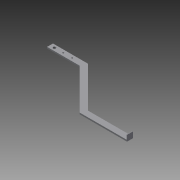
# Autodesk Inventor part: Z-PickupArm-L
Saved by Autodesk Inventor 2013 (Build 170138000, 138)
## iProperties
Created: 2014-01-22
Part Number: Z-PickupArm-L
Material: Generic
Document SubType Name: Modeling
Designer: Jarod
Density: 1 g/cm^3
Author: Jarod
Autodesk Inventor part; units mm, degrees
ref_plane "YZ Plane" through (0, 0, 0) normal (1, 0, 0) x (0, 1, 0)
ref_plane "XZ Plane" through (0, 0, 0) normal (0, 1, 0) x (-1, 0, 0)
ref_plane "XY Plane" through (0, 0, 0) normal (0, 0, 1) x (1, 0, 0)
sketch "Sketch1" plane through (0, 0, 0) normal (0, 1, 0) x (-1, 0, 0)
  line L0 (0, 0) -> (-133.35, 0)
  line L1 (-133.35, 0) -> (-133.35, 25.4)
  line L2 (-133.35, 25.4) -> (0, 25.4)
  line L3 (0, 25.4) -> (0, 0)
  line L4 (-133.35, 25.4) -> (-143.871, 0)
  line L5 (-133.35, 25.4) -> (-105.8572, 25.4) construction
  line L6 (-133.35, 25.4) -> (-151.3105, 7.4395)
  line L7 (-133.35, 25.4) -> (-107.95, 25.4) construction
  line L8 (-151.3105, 7.4395) -> (-143.871, 0)
  line L9 (-133.35, 25.4) -> (-151.3105, 7.4395)
  line L10 (-151.3105, 7.4395) -> (-318.9899, 175.1188)
  line L11 (-318.9899, 175.1188) -> (-301.0293, 193.0793)
  line L12 (-301.0293, 193.0793) -> (-133.35, 25.4)
  circle A0 centre (-12.7, 12.7) radius 6.35
  line L13 (-318.9899, 175.1188) -> (-511.6743, 175.1188)
  line L14 (-511.6743, 175.1188) -> (-511.6743, 200.5188)
  line L15 (-511.6743, 200.5188) -> (-318.9899, 200.5188)
  line L16 (-318.9899, 200.5188) -> (-318.9899, 175.1188)
  line L17 (-318.9899, 175.1188) -> (-308.4688, 200.5188)
  line L18 (-308.4688, 200.5188) -> (-318.9899, 200.5188)
  line L19 (-308.4688, 200.5188) -> (-301.0293, 193.0793)
  line L20 (-133.35, 0) -> (-143.871, 0)
  dimension "d0" = 133.35
  dimension "d1" = 25.4
  dimension "d2" = 112.5
  dimension "d3" = 25.4
  dimension "d4" = 135
  dimension "d5" = 237.1344
  dimension "d6" = 12.7
  dimension "d7" = 192.6844
  dimension "d8" = 25.4
  constraints: 42 end point, 7 parallel, 6 perpendicular, 4 horizontal, 2 equal length, 1 centre point
  measures "d0" distance of L1.end L2.end
  measures "d1" distance of L0.end L1.end
  measures "d2" angle of L4 L5
  measures "d3" distance of L1.end L6.end
  measures "d4" angle of L6 L7
  measures "d5" distance of L6.end L10.end
  measures "d6" diameter of A0
  measures "d7" distance of L14.end L15.end
  measures "d8" distance of L13.end L14.end
extrude "Extrusion1" add sketch "Sketch1" along normal blind 6.35
sketch "Sketch2" plane through (511.6743, 0, 200.5188) normal (1, 0, 0) x (0, 0, -1)
  line L0 (0, 6.35) -> (25.4, 6.35)
  line L1 (25.4, 0) -> (0, 0)
  line L2 (0, 0) -> (0, 25.4)
  line L3 (0, 25.4) -> (25.4, 25.4)
  line L4 (25.4, 25.4) -> (25.4, 0)
  point P0 (200.5188, 0)
  dimension "d15" = 25.4
  dimension "d16" = 25.4
  constraints: 10 end point, 2 horizontal, 2 parallel, 1 perpendicular
  measures "d15" distance of L2.end L3.end
  measures "d16" distance of L1.end L2.end
extrude "Extrusion2" add sketch "Sketch2" along normal blind 1.5875
sketch "Sketch3" plane through (0, 0, 0) normal (-1, 0, 0) x (0, 0, 1)
  line L0 (0, 0) -> (25.4, 0) projected
  line L1 (25.4, 0) -> (25.4, 6.35) projected
  line L2 (0, 6.35) -> (25.4, 6.35) projected
  line L3 (0, 0) -> (0, 6.35) projected
extrude "Extrusion3" add sketch "Sketch3" along normal blind 44.45
sketch "Sketch5" plane through (0, 6.35, 0) normal (0, 1, 0) x (1, 0, 0)
  circle A0 centre (12.7, -12.7) radius 6.35 projected
  line L0 (511.6743, -175.1188) -> (318.9899, -175.1188) projected
  line L1 (12.7, -12.7) -> (12.7, -6.35)
  line L2 (16.3662, -6.35) -> (20.0323, -12.7)
  line L3 (20.0323, -12.7) -> (16.3662, -19.05)
  line L4 (16.3662, -19.05) -> (9.0338, -19.05)
  line L5 (9.0338, -19.05) -> (5.3677, -12.7)
  line L6 (5.3677, -12.7) -> (9.0338, -6.35)
  line L7 (9.0338, -6.35) -> (16.3662, -6.35)
  point P0 (0, 0)
  constraints: 14 end point, 1 coincident, 1 midpoint, 1 perpendicular, 1 vertical alignment, 14 other
extrude "Extrusion5" cut sketch "Sketch5" against normal blind 6.35 contours A0 L2 L3 | A0 L7 L2 | L3 L4 A0 | A0 L6 L7 | L4 L5 A0 | A0 L5 L6
sketch "Sketch7" plane through (0, 6.35, 0) normal (0, 1, 0) x (1, 0, 0)
  line L0 (-44.45, -25.4) -> (-44.45, 0) projected
  line L1 (511.6743, -175.1188) -> (318.9899, -175.1188) projected
  line L2 (-44.45, -12.7) -> (12.7, -12.7)
  line L3 (12.7, -12.7) -> (-25.4, -12.7)
  line L4 (12.7, -12.7) -> (50.8, -12.7) construction
  line L5 (-25.4, -12.7) -> (50.8, -12.7)
  circle A0 centre (-25.4, -12.7) radius 3.175
  circle A1 centre (50.8, -12.7) radius 3.175
  point P0 (0, 0)
  dimension "d31" = 38.1
  dimension "d32" = 180
  dimension "d33" = 76.2
  dimension "d34" = 0
  dimension "d35" = 6.35
  dimension "d36" = 6.35
  constraints: 8 end point, 3 collinear, 2 centre point, 2 coincident, 1 horizontal, 1 midpoint, 1 parallel
  measures "d31" distance of L2.end L3.end
  measures "d32" angle of L3 L4
  measures "d33" distance of L3.end L5.end
  measures "d34" distance between parallel lines of L5 L3
  measures "d35" diameter of A0
  measures "d36" diameter of A1
extrude "Extrusion7" cut sketch "Sketch7" against normal blind 25.4
sketch "Sketch8" plane through (0, 6.35, 0) normal (0, 1, 0) x (1, 0, 0)
  circle A0 centre (-25.4, -12.7) radius 3.175 projected
  circle A1 centre (50.8, -12.7) radius 3.175 projected
  line L0 (-44.45, 0) -> (0, 0)
  line L1 (0, 0) -> (0, -25.4)
  line L2 (0, -25.4) -> (-44.45, -25.4)
  line L3 (-44.45, -25.4) -> (-44.45, 0)
  line L4 (0, -12.7) -> (12.7, -12.7)
  line L5 (12.7, -12.7) -> (50.8, -12.7)
  line L6 (50.8, -12.7) -> (88.9, -12.7)
  circle A2 centre (88.9, -12.7) radius 3.175
  dimension "d39" = 44.45
  dimension "d40" = 25.4
  dimension "d41" = 38.1
  dimension "d42" = 180
  dimension "d43" = 6.35
  constraints: 14 end point, 2 parallel, 2 perpendicular, 1 centre point, 1 coincident, 1 collinear, 1 horizontal, 1 midpoint
  measures "d39" distance of L1.end L2.end
  measures "d40" distance of L0.end L1.end
  measures "d41" distance of L5.end L6.end
  measures "d42" angle of L5 L6
  measures "d43" diameter of A2
extrude "Extrusion8" cut sketch "Sketch8" against normal blind 25.4 contours L1 L2 L3 L0 | A2
sketch "Sketch9" plane through (0, 6.35, 0) normal (-1, 0, 0) x (0, 0, 1)
  line L0 (25.4, -6.35) -> (0, -6.35) projected
  line L1 (25.4, 0) -> (25.4, -6.35) projected
  line L2 (0, 0) -> (25.4, 0) projected
  line L3 (0, -6.35) -> (0, 0) projected
extrude "Extrusion9" add sketch "Sketch9" along normal blind 6.35
sketch "Sketch10" plane through (0, 6.35, 0) normal (0, 1, 0) x (1, 0, 0)
  line L0 (-6.35, -25.4) -> (-6.35, 0) projected
  line L1 (5.3677, -12.7) -> (9.0338, -6.35) projected
  line L2 (9.0338, -6.35) -> (16.3662, -6.35) projected
  line L3 (16.3662, -6.35) -> (20.0323, -12.7) projected
  line L4 (20.0323, -12.7) -> (16.3662, -19.05) projected
  line L5 (16.3662, -19.05) -> (9.0338, -19.05) projected
  line L6 (9.0338, -19.05) -> (5.3677, -12.7) projected
  line L7 (-6.35, -12.7) -> (12.7, -12.7)
  line L8 (12.7, -12.7) -> (6.35, -12.7)
  line L9 (12.7, -12.7) -> (19.05, -12.7) construction
  line L10 (6.35, -12.7) -> (9.525, -7.2007)
  line L11 (9.525, -7.2007) -> (15.875, -7.2007)
  line L12 (15.875, -7.2007) -> (19.05, -12.7)
  line L13 (19.05, -12.7) -> (15.875, -18.1993)
  line L14 (15.875, -18.1993) -> (9.525, -18.1993)
  line L15 (9.525, -18.1993) -> (6.35, -12.7)
  point P0 (0, 0)
  dimension "d48" = 6.35
  dimension "d49" = 180
  constraints: 18 end point, 2 collinear, 1 coincident, 1 horizontal, 1 midpoint, 1 parallel, 13 other
  measures "d48" distance of L7.end L8.end
  measures "d49" angle of L8 L9
extrude "Extrusion10" add sketch "Sketch10" against normal blind 6.35
body "Solid1"
